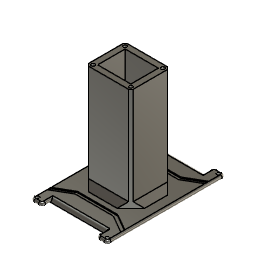
handle2 (Autodesk Fusion 360 design; units mm, degrees)
Autodesk Fusion 360 part; units mm, degrees
sketch "Sketch1" plane through (0, 0, 0) normal (0, 0, 1) x (1, 0, 0)
  line L0 (0, 0) -> (-30.625, 0)
  line L1 (0, 0) -> (30.625, 0)
  line L2 (-30.625, 0) -> (-30.625, 97)
  line L3 (-30.625, 97) -> (30.625, 97)
  line L4 (30.625, 97) -> (30.625, 0)
  circle A0 centre (-30.625, 97) radius 1.5
  circle A1 centre (30.625, 97) radius 1.5
  circle A2 centre (-30.625, 0) radius 1.5
  circle A3 centre (30.625, 0) radius 1.5
  line L5 (0, -3) -> (33.625, -3)
  line L6 (33.625, 100) -> (33.625, -3)
  line L7 (-33.625, 100) -> (33.625, 100)
  line L8 (-33.625, -3) -> (-33.625, 100)
  line L9 (0, -3) -> (-33.625, -3)
  dimension "d1" = 30.625
  dimension "d2" = 30.625
  dimension "d3" = 97
  dimension "d4" = 61.25
  dimension "d5" = 3
  dimension "d6" = 3
  dimension "d7" = 3
  dimension "d8" = 3
  dimension "d9" = -3
  constraint coincident L0.start L1.start
  constraint horizontal L0
  constraint parallel L0 L1
  constraint perpendicular L0 L2
  constraint perpendicular L2 L3
  constraint coincident L2.end L3.start
  constraint coincident L3.end L4.start
  constraint coincident L0.end L2.start
  constraint coincident L1.end L4.end
  measures "d1" distance of L0.start L0.end
  measures "d2" distance of L0.start L1.end
  measures "d3" distance of L0.end L2.end
  measures "d4" distance of L2.end L3.end
  measures "d5" diameter of A0
  measures "d6" diameter of A1
  measures "d7" diameter of A2
  measures "d8" diameter of A3
extrude "Extrude1" add sketch "Sketch1" along normal blind 3 contours L0 L1 L2 L3 L4 A0 A1 A2 A3 | L5 L6 L7 L8 L9
sketch "Sketch2" plane through (0, 0, 3) normal (0, 0, 1) x (-1, 0, 0)
  circle A0 centre (30.625, 0) radius 1.5
  circle A1 centre (30.625, -97) radius 1.5
  circle A2 centre (-30.625, 0) radius 1.5
  circle A3 centre (-30.625, -97) radius 1.5
  line L0 (33.625, 3) -> (-33.625, 3)
  line L1 (-33.625, 3) -> (-33.625, -100)
  line L2 (-33.625, -100) -> (33.625, -100)
  line L3 (33.625, -100) -> (33.625, 3)
  line L4 (14.5, -60.5) -> (-14.5, -60.5)
  circle A4 centre (-16.5, -34.5) radius 1.5
  line L5 (14.5, -36.5) -> (14.5, -60.5)
  circle A5 centre (16.5, -62.5) radius 1.5
  line L6 (-17.5, -65.5) -> (17.5, -65.5)
  line L7 (-19.5, -33.5) -> (-19.5, -63.5)
  line L8 (17.5, -65.5) -> (19.5, -63.5)
  line L9 (19.5, -63.5) -> (19.5, -33.5)
  line L10 (17.5, -31.5) -> (-17.5, -31.5)
  circle A6 centre (-16.5, -62.5) radius 1.5
  line L11 (19.5, -33.5) -> (17.5, -31.5)
  line L12 (-17.5, -31.5) -> (-19.5, -33.5)
  line L13 (-14.5, -60.5) -> (-14.5, -36.5)
  circle A7 centre (16.5, -34.5) radius 1.5
  line L14 (-19.5, -63.5) -> (-17.5, -65.5)
  line L15 (-14.5, -36.5) -> (14.5, -36.5)
  line L16 (33.625, -48.5) -> (-33.625, -48.5)
  line L17 (0, -48.5) -> (0, -70)
  point P0 (0, -48.5)
  constraint midpoint L3 L16.start
  constraint midpoint L1 L16.end
  constraint midpoint L16 P0
  constraint perpendicular L16 L17
  measures "d28" angle of L0.end
extrude "Extrude2" add sketch "Sketch2" along normal blind 90 contours L5 L7 L9 L10 L11 L12 L13 L15 L16 | L4 L5 L6 L8 L9 L16 L17 | L4 L6 L7 L13 L14 L16 L17
sketch "Sketch3" plane through (0, 0, 3) normal (0, 0, 1) x (-1, 0, 0)
  line L0 (-14.5, -60.5) -> (14.5, -60.5)
  line L1 (14.5, -60.5) -> (14.5, -36.5)
  line L2 (14.5, -36.5) -> (-14.5, -36.5)
  line L3 (-14.5, -36.5) -> (-14.5, -60.5)
  line L4 (33.625, 3) -> (-33.625, 3)
  line L5 (-33.625, 3) -> (-33.625, -100)
  line L6 (-33.625, -100) -> (33.625, -100)
  line L7 (33.625, -100) -> (33.625, 3)
  circle A0 centre (-30.625, -97) radius 1.5
  circle A1 centre (-30.625, 0) radius 1.5
  circle A2 centre (30.625, -97) radius 1.5
  circle A3 centre (30.625, 0) radius 1.5
  line L8 (-19.5, -63.5) -> (-19.5, -33.5)
  line L9 (-19.5, -33.5) -> (-17.5, -31.5)
  line L10 (-17.5, -31.5) -> (17.5, -31.5)
  line L11 (17.5, -31.5) -> (19.5, -33.5)
  line L12 (19.5, -33.5) -> (19.5, -63.5)
  line L13 (19.5, -63.5) -> (17.5, -65.5)
  line L14 (17.5, -65.5) -> (-17.5, -65.5)
  line L15 (-17.5, -65.5) -> (-19.5, -63.5)
  line L16 (30.625, 0) -> (23.625, 0)
  line L17 (23.625, 3) -> (23.625, -5)
  line L18 (-30.625, 0) -> (-23.625, 0)
  line L19 (-23.625, 3) -> (-23.625, -5)
  line L20 (23.625, -5) -> (-23.625, -5)
  line L21 (33.625, -48.5) -> (56.2227, -48.5)
  line L22 (23.625, -92) -> (-23.625, -92)
  line L23 (33.625, -100) -> (-33.625, -100)
  line L24 (23.625, -100) -> (23.625, -92)
  line L25 (-23.625, -100) -> (-23.625, -92)
  line L26 (-30.625, -97) -> (-23.625, -97)
  line L27 (30.625, -97) -> (23.625, -97)
  point P0 (0, -97)
  dimension "d14" = 7
  dimension "d15" = 8
  dimension "d16" = 7
  dimension "d17" = 8
  constraint coincident A3.centre L16.start
  constraint parallel L4 L16
  constraint coincident L4 L17.start
  constraint perpendicular L16 L17
  constraint coincident A1.centre L18.start
  constraint perpendicular L5 L18
  constraint coincident L4 L19.start
  constraint perpendicular L18 L19
  constraint midpoint L7 L21.start
  constraint perpendicular L7 L21
  constraint symmetric origin L21 P0
  constraint symmetric L4.start L21 L6.end
  constraint symmetric L4.end L21 L5.end
  constraint symmetric A3.centre L21 A2.centre
  constraint symmetric L16.end L21 L27.end
  constraint symmetric L17.start L21 L24.start
  constraint symmetric L17.end L21 L22.start
  constraint symmetric A1.centre L21 A0.centre
  constraint symmetric L18.end L21 L26.end
  constraint symmetric L19.start L21 L25.start
  constraint symmetric L19.end L21 L22.end
  measures "d14" distance of A3.centre L16.end
  measures "d15" distance of L17.start L17.end
  measures "d16" distance of A1.centre L18.end
  measures "d17" distance of L19.start L19.end
extrude "Extrude3" cut sketch "Sketch3" against normal blind 5 contours L0 L1 L2 L3 | L4 L17 L19 L20 | L6 L22 L23 L24 L25
fillet "Fillet1" radius 3 2 edges at (0, 92, 3) (0, 5, 3)
fillet "Fillet2" radius 3 8 edges at (-23.625, -3, 1.5) (-33.625, -3, 1.5) (33.625, -3, 1.5) (23.625, -3, 1.5) (-33.625, 100, 1.5) (-23.625, 100, 1.5) (23.625, 100, 1.5) (33.625, 100, 1.5)
fillet "Fillet3" radius 1.5 36 edges at (23.625, 4, 3) (24.5037, -2.1213, 3) (28.625, -3, 3) (32.7463, -2.1213, 3) (33.625, 48.5, 3) (32.7463, 99.1213, 3) (28.625, 100, 3) (24.5037, 99.1213, 3) (23.625, 93, 3) (-23.625, 93, 3) (-24.5037, 99.1213, 3) (-28.625, 100, 3) (-32.7463, 99.1213, 3) (-33.625, 48.5, 3) (-32.7463, -2.1213, 3) (-28.625, -3, 3) (-24.5037, -2.1213, 3) (-23.625, 4, 3) (23.625, 94.5, 0) (24.5037, 99.1213, 0) (28.625, 100, 0) (32.7463, 99.1213, 0) (33.625, 48.5, 0) (32.7463, -2.1213, 0) (28.625, -3, 0) (24.5037, -2.1213, 0) (23.625, 2.5, 0) (-23.625, 2.5, 0) (-24.5037, -2.1213, 0) (-28.625, -3, 0) (-32.7463, -2.1213, 0) (-33.625, 48.5, 0) (-32.7463, 99.1213, 0) (-28.625, 100, 0) (-24.5037, 99.1213, 0) (-23.625, 94.5, 0)
sketch "Sketch4" plane through (0, 0, 3) normal (0, 0, 1) x (-1, 0, 0)
  line L0 (25.125, -8) -> (-25.125, -8)
  line L1 (-25.125, -8) -> (-25.125, 0)
  arc A0 (-25.125, 0) -> (-26.625, 1.5) centre (-26.625, 0) ccw
  line L2 (-26.625, 1.5) -> (-30.625, 1.5)
  arc A1 (-32.125, 0) -> (-30.625, 1.5) centre (-30.625, 0) ccw
  line L3 (-32.125, 0) -> (-32.125, -97)
  arc A2 (-30.625, -98.5) -> (-32.125, -97) centre (-30.625, -97) ccw
  line L4 (-30.625, -98.5) -> (-26.625, -98.5)
  arc A3 (-26.625, -98.5) -> (-25.125, -97) centre (-26.625, -97) ccw
  line L5 (-25.125, -97) -> (-25.125, -89)
  line L6 (-25.125, -89) -> (25.125, -89)
  line L7 (25.125, -89) -> (25.125, -97)
  arc A4 (25.125, -97) -> (26.625, -98.5) centre (26.625, -97) ccw
  line L8 (26.625, -98.5) -> (30.625, -98.5)
  arc A5 (32.125, -97) -> (30.625, -98.5) centre (30.625, -97) ccw
  line L9 (32.125, -97) -> (32.125, 0)
  arc A6 (30.625, 1.5) -> (32.125, 0) centre (30.625, 0) ccw
  line L10 (30.625, 1.5) -> (26.625, 1.5)
  arc A7 (26.625, 1.5) -> (25.125, 0) centre (26.625, 0) ccw
  line L11 (25.125, 0) -> (25.125, -8)
  line L12 (-19.5, -63.5) -> (-19.5, -33.5)
  line L13 (-19.5, -33.5) -> (-17.5, -31.5)
  line L14 (-17.5, -31.5) -> (17.5, -31.5)
  line L15 (17.5, -31.5) -> (19.5, -33.5)
  line L16 (19.5, -33.5) -> (19.5, -63.5)
  line L17 (19.5, -63.5) -> (17.5, -65.5)
  line L18 (17.5, -65.5) -> (-17.5, -65.5)
  line L19 (-17.5, -65.5) -> (-19.5, -63.5)
  line L20 (0, -75) -> (17.5, -75)
  line L21 (17.5, -75) -> (43.5708, -90.052)
  line L22 (17.5, -75) -> (47.604, -75) construction
  line L23 (32.125, -48.5) -> (46.4762, -48.5)
  line L24 (-17.5, -75) -> (-43.5708, -90.052)
  line L25 (0, -75) -> (-17.5, -75)
  line L26 (16.6962, -78) -> (42.0708, -92.6501)
  line L27 (0, -78) -> (16.6962, -78)
  line L28 (0, -78) -> (-16.6962, -78)
  line L29 (-16.6962, -78) -> (-42.0708, -92.6501)
  line L30 (16.6962, -19) -> (42.0708, -4.3499)
  line L31 (17.5, -22) -> (43.5708, -6.948)
  line L32 (0, -22) -> (17.5, -22)
  line L33 (0, -19) -> (16.6962, -19)
  line L34 (-16.6962, -19) -> (-42.0708, -4.3499)
  line L35 (-17.5, -22) -> (-43.5708, -6.948)
  line L36 (0, -22) -> (-17.5, -22)
  line L37 (0, -19) -> (-16.6962, -19)
  line L38 (33.625, 0) -> (32.125, 0)
  line L39 (32.125, 0) -> (32.125, -97)
  line L40 (32.125, -97) -> (33.625, -97)
  line L41 (32.125, -97) -> (32.125, 0)
  line L42 (32.125, -97) -> (33.625, -97)
  arc A8 (30.625, -98.5) -> (32.125, -97) centre (30.625, -97) ccw
  line L43 (30.625, -100) -> (30.625, -98.5)
  arc A9 (30.625, -98.5) -> (32.125, -97) centre (30.625, -97) ccw
  line L44 (30.625, -100) -> (30.625, -98.5)
  line L45 (30.625, -98.5) -> (26.625, -98.5)
  line L46 (26.625, -98.5) -> (26.625, -100)
  line L47 (26.625, -98.5) -> (30.625, -98.5)
  line L48 (26.625, -98.5) -> (26.625, -100)
  arc A10 (25.125, -97) -> (26.625, -98.5) centre (26.625, -97) ccw
  line L49 (23.625, -97) -> (25.125, -97)
  arc A11 (25.125, -97) -> (26.625, -98.5) centre (26.625, -97) ccw
  line L50 (23.625, -97) -> (25.125, -97)
  line L51 (25.125, -97) -> (25.125, -89)
  spline S0 degree 3 poles (23.625, -91.5981) (23.625, -91.4847) (23.6653, -91.3409) (23.8021, -91.0199) (23.898, -90.8428) (24.1441, -90.426) (24.329, -90.1444) (24.7236, -89.5673) (24.9329, -89.2716) (25.125, -89) knots 0.801784 0.801784 0.801784 0.801784 0.869795 0.869795 0.937806 0.937806 1.037599 1.037599 1.137392 1.137392 1.137392 1.137392
  spline S1 degree 3 poles (25.125, -92) (24.9363, -92) (24.7352, -92.0007) (24.3655, -91.9949) (24.197, -91.9873) (23.9239, -91.9469) (23.8064, -91.9096) (23.6572, -91.7856) (23.625, -91.6979) (23.625, -91.5981) knots 0.568638 0.568638 0.568638 0.568638 0.625237 0.625237 0.681836 0.681836 0.741752 0.741752 0.801668 0.801668 0.801668 0.801668
  line L52 (25.125, -92) -> (25.125, -97)
  line L53 (-25.125, -92) -> (25.125, -92)
  spline S2 degree 3 poles (25.125, -92) (24.9363, -92) (24.7352, -92.0007) (24.3655, -91.9949) (24.197, -91.9873) (23.9239, -91.9469) (23.8064, -91.9096) (23.6572, -91.7856) (23.625, -91.6979) (23.625, -91.5981) knots 0.568638 0.568638 0.568638 0.568638 0.625237 0.625237 0.681836 0.681836 0.741752 0.741752 0.801668 0.801668 0.801668 0.801668
  spline S3 degree 3 poles (23.625, -91.5981) (23.625, -91.4847) (23.6653, -91.3409) (23.8021, -91.0199) (23.898, -90.8428) (24.1441, -90.426) (24.329, -90.1444) (24.7236, -89.5673) (24.9329, -89.2716) (25.125, -89) knots 0.801784 0.801784 0.801784 0.801784 0.869795 0.869795 0.937806 0.937806 1.037599 1.037599 1.137392 1.137392 1.137392 1.137392
  line L54 (25.125, -89) -> (-25.125, -89)
  spline S4 degree 3 poles (-25.125, -89) (-24.9329, -89.2716) (-24.7236, -89.5673) (-24.329, -90.1444) (-24.1441, -90.426) (-23.898, -90.8428) (-23.8021, -91.0199) (-23.6653, -91.3409) (-23.625, -91.4847) (-23.625, -91.5981) knots 0 0 0 0 0.099793 0.099793 0.199586 0.199586 0.267597 0.267597 0.335608 0.335608 0.335608 0.335608
  spline S5 degree 3 poles (-23.625, -91.5981) (-23.625, -91.6979) (-23.6572, -91.7856) (-23.8064, -91.9096) (-23.9239, -91.9469) (-24.197, -91.9873) (-24.3655, -91.9949) (-24.7352, -92.0007) (-24.9363, -92) (-25.125, -92) knots 0.335608 0.335608 0.335608 0.335608 0.395524 0.395524 0.455441 0.455441 0.512039 0.512039 0.568638 0.568638 0.568638 0.568638
  line L55 (30.625, 1.5) -> (30.625, 3)
  arc A12 (32.125, 0) -> (30.625, 1.5) centre (30.625, 0) ccw
  line L56 (33.625, 0) -> (32.125, 0)
  arc A13 (32.125, 0) -> (30.625, 1.5) centre (30.625, 0) ccw
  line L57 (26.625, 3) -> (26.625, 1.5)
  line L58 (26.625, 1.5) -> (30.625, 1.5)
  line L59 (30.625, 1.5) -> (30.625, 3)
  line L60 (30.625, 1.5) -> (26.625, 1.5)
  line L61 (25.125, 0) -> (23.625, 0)
  arc A14 (26.625, 1.5) -> (25.125, 0) centre (26.625, 0) ccw
  line L62 (26.625, 3) -> (26.625, 1.5)
  arc A15 (26.625, 1.5) -> (25.125, 0) centre (26.625, 0) ccw
  spline S6 degree 3 poles (25.125, -8) (24.9329, -7.7284) (24.7236, -7.4327) (24.329, -6.8556) (24.1441, -6.574) (23.898, -6.1572) (23.8021, -5.9801) (23.6653, -5.6591) (23.625, -5.5153) (23.625, -5.4019) knots 0 0 0 0 0.099793 0.099793 0.199586 0.199586 0.267597 0.267597 0.335608 0.335608 0.335608 0.335608
  line L63 (25.125, -8) -> (25.125, 0)
  line L64 (25.125, 0) -> (23.625, 0)
  line L65 (25.125, 0) -> (25.125, -5)
  spline S7 degree 3 poles (23.625, -5.4019) (23.625, -5.3021) (23.6572, -5.2144) (23.8064, -5.0904) (23.9239, -5.0531) (24.197, -5.0127) (24.3655, -5.0051) (24.7352, -4.9993) (24.9363, -5) (25.125, -5) knots 0.335608 0.335608 0.335608 0.335608 0.395524 0.395524 0.455441 0.455441 0.512039 0.512039 0.568638 0.568638 0.568638 0.568638
  line L66 (25.125, -5) -> (-25.125, -5)
  spline S8 degree 3 poles (-25.125, -5) (-24.9363, -5) (-24.7352, -4.9993) (-24.3655, -5.0051) (-24.197, -5.0127) (-23.9239, -5.0531) (-23.8064, -5.0904) (-23.6572, -5.2144) (-23.625, -5.3021) (-23.625, -5.4019) knots 0.568638 0.568638 0.568638 0.568638 0.625237 0.625237 0.681836 0.681836 0.741752 0.741752 0.801668 0.801668 0.801668 0.801668
  spline S9 degree 3 poles (-23.625, -5.4019) (-23.625, -5.5153) (-23.6653, -5.6591) (-23.8021, -5.9801) (-23.898, -6.1572) (-24.1441, -6.574) (-24.329, -6.8556) (-24.7236, -7.4327) (-24.9329, -7.7284) (-25.125, -8) knots 0.801668 0.801668 0.801668 0.801668 0.869679 0.869679 0.93769 0.93769 1.037483 1.037483 1.137277 1.137277 1.137277 1.137277
  line L67 (-25.125, -8) -> (25.125, -8)
  spline S10 degree 3 poles (25.125, -8) (24.9329, -7.7284) (24.7236, -7.4327) (24.329, -6.8556) (24.1441, -6.574) (23.898, -6.1572) (23.8021, -5.9801) (23.6653, -5.6591) (23.625, -5.5153) (23.625, -5.4019) knots 0 0 0 0 0.099793 0.099793 0.199586 0.199586 0.267597 0.267597 0.335608 0.335608 0.335608 0.335608
  spline S11 degree 3 poles (23.625, -5.4019) (23.625, -5.3021) (23.6572, -5.2144) (23.8064, -5.0904) (23.9239, -5.0531) (24.197, -5.0127) (24.3655, -5.0051) (24.7352, -4.9993) (24.9363, -5) (25.125, -5) knots 0.335608 0.335608 0.335608 0.335608 0.395524 0.395524 0.455441 0.455441 0.512039 0.512039 0.568638 0.568638 0.568638 0.568638
  line L68 (-33.625, -97) -> (-32.125, -97)
  line L69 (-32.125, -97) -> (-32.125, 0)
  line L70 (-32.125, 0) -> (-33.625, 0)
  line L71 (-32.125, 0) -> (-32.125, -97)
  dimension "d27" = 17.5
  dimension "d28" = 30
  dimension "d29" = -3
  constraint horizontal L22
  constraint midpoint L9 L23.start
  constraint perpendicular L9 L23
  constraint symmetric L20.start L23 L32.start
  constraint symmetric L20.end L23 L31.start
  constraint symmetric L21.end L23 L31.end
  constraint symmetric L23 L24.start L35.start
  constraint symmetric L23 L24.end L35.end
  constraint symmetric L23 L20.start L32.start
  constraint symmetric L23 L26.start L30.start
  constraint symmetric L23 L26.end L30.end
  constraint symmetric L23 L27.start L33.start
  constraint symmetric L23 L28.end L34.start
  constraint symmetric L23 L29.end L34.end
  measures "d27" distance of L20.start L20.end
  measures "d28" angle of L21 L22
extrude "Extrude4" cut sketch "Sketch4" against normal blind 1 contours L3 L9 L30 L31 L32 L33 L34 L35 L36 L37 L39 L41 L69 L71 | L3 L9 L20 L21 L24 L25 L26 L27 L28 L29 L39 L41 L69 L71
chamfer "Chamfer1" distance 5 angle 45 4 edges at (0, 31.5, 3) (0, 65.5, 3) (19.5, 48.5, 3) (-19.5, 48.5, 3)
